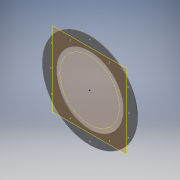
# Autodesk Inventor part: Ring Gear Outer
Saved by Autodesk Inventor 2016 (Build 200138000, 138)
## iProperties
Created: 2016-04-25
Part Number: Ring Gear Outer
Material: Generic
Document SubType Name: Modeling
Designer: rubenjm
Density: 1 g/cm^3
Appearance: Default
Author: rubenjm
Autodesk Inventor part; units mm, degrees
ref_plane "YZ Plane" through (0, 0, 0) normal (1, 0, 0) x (0, 1, 0)
ref_plane "XZ Plane" through (0, 0, 0) normal (0, 1, 0) x (-1, 0, 0)
ref_plane "XY Plane" through (0, 0, 0) normal (0, 0, 1) x (1, 0, 0)
sketch "Sketch1" plane through (0, 0, 0) normal (0, 0, 1) x (1, 0, 0)
  circle A0 centre (0, 0) radius 136.271
  circle A1 centre (0, 0) radius 190.5
  dimension "d0" = 272.542
  dimension "d1" = 381
  constraints: 2 centre point, 2 coincident
  measures "d0" diameter of A0
  measures "d1" diameter of A1
extrude "Extrusion1" add sketch "Sketch1" against normal blind 3.175
sketch "Sketch2" plane through (0, 0, 0) normal (0, 0, 1) x (1, 0, 0)
  circle A0 centre (0, 0) radius 157.48 construction
  circle A1 centre (-157.48, 0) radius 3.9687
  circle A2 centre (-78.74, -136.3817) radius 3.9687
  circle A3 centre (78.74, -136.3817) radius 3.9687
  circle A4 centre (157.48, 0) radius 3.9687
  circle A5 centre (78.74, 136.3817) radius 3.9687
  circle A6 centre (-78.74, 136.3817) radius 3.9687
  dimension "d6" = 314.96
  dimension "d7" = 7.9375
  dimension "d8" = 360
  constraints: 6 centre point, 1 coincident, 1 horizontal alignment, 15 other
  measures "d7" diameter of A1
extrude "Extrusion2" cut sketch "Sketch2" against normal through all
sketch "Sketch3" plane through (0, 0, 0) normal (0, 0, 1) x (1, 0, 0)
  line L0 (0, 0) -> (0, -177.8) construction
  line L1 (0, 0) -> (177.8, 0) construction
  circle A0 centre (0, -177.8) radius 3.81
  circle A1 centre (153.9793, -88.9) radius 3.81
  circle A2 centre (153.9793, 88.9) radius 3.81
  circle A3 centre (0, 177.8) radius 3.81
  circle A4 centre (-153.9793, 88.9) radius 3.81
  circle A5 centre (-153.9793, -88.9) radius 3.81
  line L2 (0, 0) -> (0, -177.8) construction
  line L3 (0, 0) -> (177.8, 0) construction
  circle A6 centre (0, -177.8) radius 3.81
  circle A7 centre (153.9793, -88.9) radius 3.81
  circle A8 centre (153.9793, 88.9) radius 3.81
  circle A9 centre (0, 177.8) radius 3.81
  circle A10 centre (-153.9793, 88.9) radius 3.81
  circle A11 centre (-153.9793, -88.9) radius 3.81
  line L4 (0, 0) -> (0, -177.8) construction
  line L5 (0, 0) -> (177.8, 0) construction
  circle A12 centre (0, -177.8) radius 3.81
  circle A13 centre (153.9793, -88.9) radius 3.81
  circle A14 centre (153.9793, 88.9) radius 3.81
  circle A15 centre (0, 177.8) radius 3.81
  circle A16 centre (-153.9793, 88.9) radius 3.81
  circle A17 centre (-153.9793, -88.9) radius 3.81
  dimension "d13" = 177.8
  dimension "d14" = 90
  dimension "d15" = 7.62
  dimension "d16" = 360
  dimension "d19" = 177.8
  dimension "d20" = 90
  dimension "d21" = 7.62
  dimension "d22" = 360
  dimension "d25" = 177.8
  dimension "d26" = 90
  dimension "d27" = 7.62
  dimension "d28" = 360
  constraints: 18 centre point, 12 end point, 3 coincident, 3 horizontal, 3 perpendicular, 3 vertical, 39 other
  measures "d13" distance of L0.start L0.end
  measures "d14" angle of L0 L1
  measures "d15" diameter of A0
  measures "d19" distance of L2.start L2.end
  measures "d20" angle of L2 L3
  measures "d21" diameter of A6
  measures "d25" distance of L4.start L4.end
  measures "d26" angle of L4 L5
  measures "d27" diameter of A12
extrude "Extrusion3" cut sketch "Sketch3" against normal through all
ref_plane "Work Plane1" through (0, 0, 0) normal (0, 0, 1) x (1, 0, 0)
sketch "Sketch4" plane through (0, 0, 0) normal (0, 0, 1) x (1, 0, 0)
  circle A0 centre (0, 0) radius 124.1061 construction
  constraints: 1 centre point, 1 coincident
body "Solid1"
